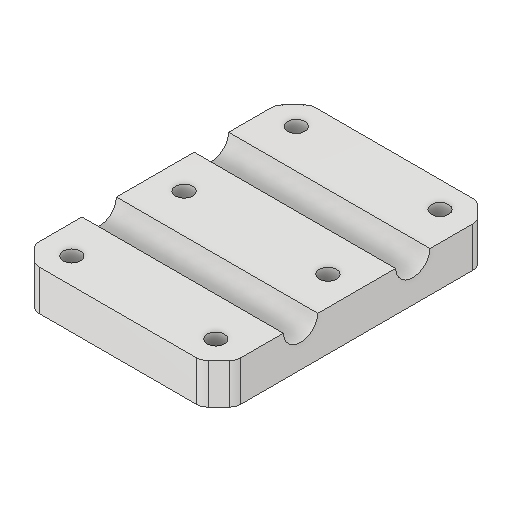
# Autodesk Inventor part: 3DP_PLA_X_end_top_linear_shaft_clamp
Saved by Autodesk Inventor 2026.1 (Build 301233000, 233)
## iProperties
Created: 2018-07-03
Part Number: 3DP_PLA_X_end_top_linear_shaft_clamp
Material: ABS Plastic
Document SubType Name: Modeling
Designer: Andrzej
Density: 1.06 g/cm^3
Appearance: Smooth - White
Author: Andrzej
Autodesk Inventor part; units mm, degrees
ref_plane "YZ Plane" through (0, 0, 0) normal (1, 0, 0) x (0, 1, 0)
ref_plane "XZ Plane" through (0, 0, 0) normal (0, 1, 0) x (-1, 0, 0)
ref_plane "XY Plane" through (0, 0, 0) normal (0, 0, 1) x (1, 0, 0)
sketch "Sketch1" plane through (0, 0, 0) normal (0, 0, 1) x (1, 0, 0)
  line L0 (-17.4973, 3.5) -> (-17.4973, 10.5)
  line L1 (-17.4973, 10.5) -> (17.5027, 10.5)
  line L2 (17.5027, 10.5) -> (17.5027, 3.5)
  line L3 (-17.4973, 3.5) -> (17.5027, 3.5)
  dimension "d50" = 35
  dimension "d51" = 7
  constraints: 8 end point, 2 horizontal, 1 perpendicular, 1 vertical
  measures "d50" distance of L0.end L1.end
  measures "d51" distance of L0.start L0.end
extrude "Extrusion1" add sketch "Sketch1" along normal blind 48
sketch "Sketch4" plane through (-17.4973, 3.5, 0) normal (0, -1, 0) x (1, 0, 0)
  line L0 (35, 0) -> (0, 0) projected
  line L1 (35, 0) -> (35, 48) projected
  line L2 (0, 48) -> (35, 48) projected
  line L3 (0, 0) -> (0, 48) projected
  point P0 (5, 4.5)
  point P1 (5, 24)
  point P2 (5, 43.5)
  point P3 (30, 4.5)
  point P4 (30, 24)
  point P5 (30, 43.5)
  dimension "d52" = 4.5
  dimension "d53" = 4.5
  dimension "d54" = 5
  dimension "d55" = 5
  dimension "d56" = 24
  constraints: 4 vertical alignment, 3 horizontal alignment
  measures "d52" distance from line of L0 point (5, 4.5)
  measures "d53" distance from line of L2 point (5, 43.5)
  measures "d54" distance from line of L3 point (5, 4.5)
  measures "d55" distance from line of L1 point (30, 4.5)
  measures "d56" distance from line of L0 point (5, 24)
hole "Hole2" at (-12.4973, 3.5, 4.5) at (-12.4973, 3.5, 24) at (-12.4973, 3.5, 43.5) at (12.5027, 3.5, 4.5) at (12.5027, 3.5, 24) at (12.5027, 3.5, 43.5) direction (0, 1, 0) diameter 3 end through all
sketch "Sketch5" plane through (17.5027, 3.5, 0) normal (1, 0, 0) x (0, 0, -1)
  circle A0 centre (-14.25, 7.1) radius 3
  circle A1 centre (-33.75, 7.1) radius 3
  line L0 (0, 7) -> (0, 0) projected
  line L1 (0, 7) -> (-48, 7) projected
  line L2 (-48, 0) -> (-48, 7) projected
  line L3 (0, 0) -> (-48, 0) projected
  point P0 (0, -3.5)
  dimension "d64" = 6
  dimension "d65" = 6
  dimension "d66" = 0.1
  dimension "d67" = 0.1
  dimension "d68" = 14.25
  dimension "d69" = 14.25
  constraints: 2 centre point
  measures "d64" diameter of A0
  measures "d65" diameter of A1
  measures "d66" distance from line of L1 A0.centre
  measures "d67" distance from line of L1 A1.centre
  measures "d68" distance from line of A0.centre L0
  measures "d69" distance from line of L2 A1.centre
extrude "Extrusion3" cut sketch "Sketch5" against normal up to next contours A0 L1 | L1 A0 | L1 A1 | A1 L1
chamfer "Chamfer1" distance 3 angle 45 4 edges at (-17.4973, 7, 0) (-17.4973, 7, 48) (17.5027, 7, 48) (17.5027, 7, 0)
fillet "Fillet2" radius 2 8 edges at (-17.4973, 7, 3) (-14.4973, 7, 0) (-17.4973, 7, 45) (-14.4973, 7, 48) (14.5027, 7, 48) (17.5027, 7, 45) (14.5027, 7, 0) (17.5027, 7, 3)
equation "\"d53\" = d52"
equation "\"d55\" = d54"
equation "\"d69\" = d68"
body "Solid1"
